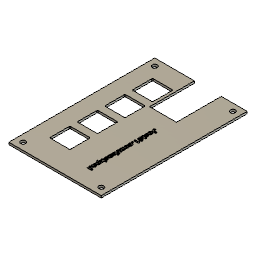
Hackpad Top v1 (Autodesk Fusion 360 design; units mm, degrees)
Autodesk Fusion 360 part; units mm, degrees
sketch "Sketch1" plane through (0, 0, 0) normal (0, 1, 0) x (1, 0, 0)
  line L0 (32, 50.5) -> (-32, 50.5)
  line L1 (-32, 50.5) -> (-32, -50.5)
  line L2 (-32, -50.5) -> (32, -50.5)
  line L3 (32, -50.5) -> (32, 50.5)
  line L4 (32, 50.5) -> (-32, -50.5) construction
  line L5 (-32, 50.5) -> (32, -50.5) construction
  line L6 (-22, 40.5) -> (22, -40.5) construction
  line L7 (14, 40.5) -> (14, 50.5)
  line L8 (14, 50.5) -> (22, 50.5)
  line L9 (14, 50.5) -> (-4.5, 50.5)
  line L10 (-4.5, 50.5) -> (-4.5, 19.5)
  line L11 (-4.5, 19.5) -> (14, 19.5)
  line L12 (14, 19.5) -> (14, 50.5)
  line L13 (32, 50.5) -> (27, 50.5)
  line L14 (32, 45.5) -> (32, 50.5)
  line L15 (-32, 50.5) -> (-27, 50.5)
  line L16 (-32, 45.5) -> (-32, 50.5)
  line L17 (-32, -50.5) -> (-27, -50.5)
  line L18 (-32, -45.5) -> (-32, -50.5)
  line L19 (32, -50.5) -> (27, -50.5)
  line L20 (32, -45.5) -> (32, -50.5)
  circle A0 centre (-27, 45.5) radius 1.7
  circle A1 centre (27, 45.5) radius 1.7
  circle A2 centre (27, -45.5) radius 1.7
  line L21 (-19.975, 37.475) -> (-6.975, 37.475)
  line L22 (-19.975, 23.475) -> (-6.975, 23.475)
  line L23 (-20.475, 36.975) -> (-20.475, 23.975)
  line L24 (-6.475, 36.975) -> (-6.475, 23.975)
  arc A3 (-19.975, 37.475) -> (-20.475, 36.975) centre (-19.975, 36.975) ccw
  arc A4 (-6.475, 36.975) -> (-6.975, 37.475) centre (-6.975, 36.975) ccw
  arc A5 (-20.475, 23.975) -> (-19.975, 23.475) centre (-19.975, 23.975) ccw
  arc A6 (-6.975, 23.475) -> (-6.475, 23.975) centre (-6.975, 23.975) ccw
  line L25 (-19.975, 18.425) -> (-6.975, 18.425)
  line L26 (-19.975, 4.425) -> (-6.975, 4.425)
  line L27 (-20.475, 17.925) -> (-20.475, 4.925)
  line L28 (-6.475, 17.925) -> (-6.475, 4.925)
  arc A7 (-19.975, 18.425) -> (-20.475, 17.925) centre (-19.975, 17.925) ccw
  arc A8 (-6.475, 17.925) -> (-6.975, 18.425) centre (-6.975, 17.925) ccw
  arc A9 (-20.475, 4.925) -> (-19.975, 4.425) centre (-19.975, 4.925) ccw
  arc A10 (-6.975, 4.425) -> (-6.475, 4.925) centre (-6.975, 4.925) ccw
  line L29 (-19.975, -0.625) -> (-6.975, -0.625)
  line L30 (-19.975, -14.625) -> (-6.975, -14.625)
  line L31 (-20.475, -1.125) -> (-20.475, -14.125)
  line L32 (-6.475, -1.125) -> (-6.475, -14.125)
  arc A11 (-19.975, -0.625) -> (-20.475, -1.125) centre (-19.975, -1.125) ccw
  arc A12 (-6.475, -1.125) -> (-6.975, -0.625) centre (-6.975, -1.125) ccw
  arc A13 (-20.475, -14.125) -> (-19.975, -14.625) centre (-19.975, -14.125) ccw
  arc A14 (-6.975, -14.625) -> (-6.475, -14.125) centre (-6.975, -14.125) ccw
  line L33 (-19.975, -19.675) -> (-6.975, -19.675)
  line L34 (-19.975, -33.675) -> (-6.975, -33.675)
  line L35 (-20.475, -20.175) -> (-20.475, -33.175)
  line L36 (-6.475, -20.175) -> (-6.475, -33.175)
  arc A15 (-19.975, -19.675) -> (-20.475, -20.175) centre (-19.975, -20.175) ccw
  arc A16 (-6.475, -20.175) -> (-6.975, -19.675) centre (-6.975, -20.175) ccw
  arc A17 (-20.475, -33.175) -> (-19.975, -33.675) centre (-19.975, -33.175) ccw
  arc A18 (-6.975, -33.675) -> (-6.475, -33.175) centre (-6.975, -33.175) ccw
  circle A19 centre (-27, -45.5) radius 1.7
  dimension "d1" = 64
  dimension "d2" = 101
  dimension "d6" = 18.5
  dimension "d7" = 31
  dimension "d8" = 5
  dimension "d9" = 5
  dimension "d10" = 5
  dimension "d11" = 5
  dimension "d12" = 5
  dimension "d13" = 5
  dimension "d14" = 5
  dimension "d15" = 5
  dimension "d16" = 3.4
  dimension "d17" = 3.4
  dimension "d18" = 3.4
  dimension "d19" = 3.4
  constraint horizontal L0
  constraint perpendicular L0 L1
  constraint parallel L0 L2
  constraint parallel L1 L3
  constraint coincident L4 origin
  constraint coincident L5 origin
  constraint coincident L6 origin
  constraint vertical L7
  constraint horizontal L8
  constraint horizontal L9
  constraint vertical L10
  constraint horizontal L11
  constraint vertical L12
  constraint horizontal L13
  constraint vertical L14
  constraint horizontal L15
  constraint vertical L16
  constraint horizontal L17
  constraint vertical L18
  constraint horizontal L19
  constraint vertical L20
  measures "d1" distance of L1.end L2.end
  measures "d2" distance of L0.end L1.end
  measures "d6" distance of L7.end L9.end
  measures "d7" distance of L7.end L11.end
  measures "d8" distance of L0.start L13.end
  measures "d9" distance of L0.start L14.start
  measures "d10" distance of L0.end L15.end
  measures "d11" distance of L0.end L16.start
  measures "d12" distance of L1.end L17.end
  measures "d13" distance of L1.end L18.start
  measures "d14" distance of L2.end L19.end
  measures "d15" distance of L2.end L20.start
  measures "d16" diameter of A0
  measures "d17" diameter of A1
  measures "d18" diameter of A2
  measures "d19" diameter of A19
extrude "Extrude1" add sketch "Sketch1" along normal blind 1.5 contours L0 L1 L2 L3 L7 L8 L10 L11 L12 L13 L14 L15 L16 L17 L18 L19 L20
sketch "Sketch2" plane through (0, 1.5, 0) normal (0, 1, 0) x (-1, 0, 0)
  circle A0 centre (27, 45.5) radius 1.7
  arc A1 (19.975, 19.675) -> (20.475, 20.175) centre (19.975, 20.175) ccw
  line L0 (19.975, 19.675) -> (6.975, 19.675)
  arc A2 (6.475, 20.175) -> (6.975, 19.675) centre (6.975, 20.175) ccw
  line L1 (6.475, 20.175) -> (6.475, 33.175)
  arc A3 (6.975, 33.675) -> (6.475, 33.175) centre (6.975, 33.175) ccw
  line L2 (6.975, 33.675) -> (19.975, 33.675)
  arc A4 (20.475, 33.175) -> (19.975, 33.675) centre (19.975, 33.175) ccw
  line L3 (20.475, 33.175) -> (20.475, 20.175)
  circle A5 centre (-27, -45.5) radius 1.7
  circle A6 centre (-27, 45.5) radius 1.7
  arc A7 (19.975, -18.425) -> (20.475, -17.925) centre (19.975, -17.925) ccw
  line L4 (19.975, -18.425) -> (6.975, -18.425)
  arc A8 (6.475, -17.925) -> (6.975, -18.425) centre (6.975, -17.925) ccw
  line L5 (6.475, -17.925) -> (6.475, -4.925)
  arc A9 (6.975, -4.425) -> (6.475, -4.925) centre (6.975, -4.925) ccw
  line L6 (6.975, -4.425) -> (19.975, -4.425)
  arc A10 (20.475, -4.925) -> (19.975, -4.425) centre (19.975, -4.925) ccw
  line L7 (20.475, -4.925) -> (20.475, -17.925)
  arc A11 (19.975, 0.625) -> (20.475, 1.125) centre (19.975, 1.125) ccw
  line L8 (19.975, 0.625) -> (6.975, 0.625)
  arc A12 (6.475, 1.125) -> (6.975, 0.625) centre (6.975, 1.125) ccw
  line L9 (6.475, 1.125) -> (6.475, 14.125)
  arc A13 (6.975, 14.625) -> (6.475, 14.125) centre (6.975, 14.125) ccw
  line L10 (6.975, 14.625) -> (19.975, 14.625)
  arc A14 (20.475, 14.125) -> (19.975, 14.625) centre (19.975, 14.125) ccw
  line L11 (20.475, 14.125) -> (20.475, 1.125)
  circle A15 centre (27, -45.5) radius 1.7
  arc A16 (19.975, -37.475) -> (20.475, -36.975) centre (19.975, -36.975) ccw
  line L12 (19.975, -37.475) -> (6.975, -37.475)
  arc A17 (6.475, -36.975) -> (6.975, -37.475) centre (6.975, -36.975) ccw
  line L13 (6.475, -36.975) -> (6.475, -23.975)
  arc A18 (6.975, -23.475) -> (6.475, -23.975) centre (6.975, -23.975) ccw
  line L14 (6.975, -23.475) -> (19.975, -23.475)
  arc A19 (20.475, -23.975) -> (19.975, -23.475) centre (19.975, -23.975) ccw
  line L15 (20.475, -23.975) -> (20.475, -36.975)
  line L16 (-32, 50.5) -> (-32, -50.5)
  line L17 (-32, -50.5) -> (-14, -50.5)
  line L18 (-14, -50.5) -> (-14, -19.5)
  line L19 (-14, -19.5) -> (4.5, -19.5)
  line L20 (4.5, -19.5) -> (4.5, -50.5)
  line L21 (4.5, -50.5) -> (32, -50.5)
  line L22 (32, -50.5) -> (32, 50.5)
  line L23 (32, 50.5) -> (-32, 50.5)
  line L24 (-2.3629, -13.6709) -> (-2.3629, 44.0508) construction
  line L25 (-2.3629, 44.0508) -> (-21.2659, 44.0508) construction
  line L26 (-21.2659, 44.0508) -> (-21.2659, -13.6709) construction
  line L27 (-21.2659, -13.6709) -> (-2.3629, -13.6709) construction
  dimension "d22" = 3
  dimension "d23" = 0
  text T0 "Joshi1.com/hackpad" font "Arial Black" height 3 align centre middle in box 57.7217 x 18.903 at (-2.3629, -13.6709) x (0, 1) y (-1, 0) spacing 1
extrude "Extrude2" cut sketch "Sketch2" against normal blind 0.2 text T0
equation "d23 = 'Joshi1.com/hackpad'"
